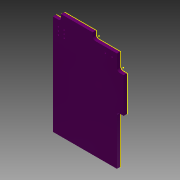
# Autodesk Inventor part: BarePCB
Saved by Autodesk Inventor 2015 SP2 (Build 190223200, 223)
## iProperties
Created: 2016-07-13
Part Number: BarePCB
Material: Generic
Document SubType Name: Modeling
Designer: Iain
Density: 1 g/cm^3
Appearance: Default
Mass: 2.23932 g
Surface Area: 30.5236 cm^2
Volume: 2.23932 cm^3
Author: Iain
Autodesk Inventor part; units mm, degrees
ref_plane "YZ Plane" through (0, 0, 0) normal (1, 0, 0) x (0, 1, 0)
ref_plane "XZ Plane" through (0, 0, 0) normal (0, 1, 0) x (-1, 0, 0)
ref_plane "XY Plane" through (0, 0, 0) normal (0, 0, 1) x (1, 0, 0)
sketch "Sketch1" plane through (0, 0, 0) normal (0, 1, 0) x (-1, 0, 0)
  line L0 (14.5, -22.6) -> (-14.5, -22.6)
  line L1 (-14.5, -22.6) -> (-14.5, 22.6)
  line L2 (-14.5, 22.6) -> (14.5, 22.6)
  line L3 (14.5, 22.6) -> (14.5, -22.6)
  point P0 (0, 0)
  point P1 (0, -22.6)
  point P2 (14.5, 0)
  dimension "d0" = 29
  dimension "d1" = 45.2
  constraints: 8 end point, 2 midpoint, 2 parallel, 1 horizontal, 1 horizontal alignment, 1 perpendicular, 1 vertical alignment
  measures "d0" distance of L0.start L0.end
  measures "d1" distance of L0.end L1.end
extrude "Extrusion1" add sketch "Sketch1" along normal blind 1.6
sketch "Sketch2" plane through (0, 1.6, 0) normal (0, 1, 0) x (1, 0, 0)
  line L0 (14.5, 22.6) -> (-14.5, 22.6) projected
  line L1 (-14.5, 22.6) -> (-14.5, -22.6) projected
  line L2 (-14.5, -22.6) -> (14.5, -22.6) projected
  line L3 (14.5, -22.6) -> (14.5, 22.6) projected
  line L4 (14.5, 0.35) -> (17.5, 0.35)
  line L5 (17.5, 0.35) -> (17.5, -15.6)
  line L6 (17.5, -15.6) -> (14.5, -15.6)
  line L7 (14.5, -15.6) -> (14.5, 0.35)
  point P0 (0, 0)
  point P1 (14.5, -7.625)
  point P2 (14.5, 0)
  dimension "d4" = 3
  dimension "d5" = 15.95
  dimension "d6" = 7
  constraints: 8 end point, 2 midpoint, 2 parallel, 1 horizontal, 1 perpendicular, 1 vertical alignment
  measures "d4" distance of L4.start L4.end
  measures "d5" distance of L4.end L5.end
  measures "d6" distance between parallel lines of L2 L6
extrude "Extrusion2" add sketch "Sketch2" against normal up to surface (1.6 mm away) contours L4 L5 L6 L3
sketch "Sketch3" plane through (0, 1.6, 0) normal (0, 1, 0) x (1, 0, 0)
  line L0 (14.5, 22.6) -> (-14.5, 22.6) projected
  line L1 (-14.5, 22.6) -> (-14.5, -22.6) projected
  line L2 (-14.5, -22.6) -> (14.5, -22.6) projected
  line L3 (14.5, -22.6) -> (14.5, -15.6) projected
  line L4 (17.5, -15.6) -> (14.5, -15.6) projected
  line L5 (17.5, 0.35) -> (17.5, -15.6) projected
  line L6 (14.5, 0.35) -> (17.5, 0.35) projected
  line L7 (14.5, 0.35) -> (14.5, 22.6) projected
  line L8 (-10.8, -22.6) -> (3.5, -22.6)
  line L9 (3.5, -22.6) -> (3.5, -25.4)
  line L10 (3.5, -25.4) -> (-10.8, -25.4)
  line L11 (-10.8, -25.4) -> (-10.8, -22.6)
  line L12 (-14.5, -22.6) -> (14.5, -22.6) projected
  point P0 (0, 0)
  point P1 (-3.65, -22.6)
  point P2 (0, -22.6)
  dimension "d9" = 2.8
  dimension "d10" = 14.3
  dimension "d11" = 3.7
  constraints: 8 end point, 2 midpoint, 2 parallel, 1 horizontal, 1 horizontal alignment, 1 perpendicular
  measures "d9" distance of L8.end L9.end
  measures "d10" distance of L9.end L10.end
  measures "d11" distance between parallel lines of L11 L1
extrude "Extrusion3" add sketch "Sketch3" against normal up to surface (1.6 mm away) contours L2 L9 L10 L11
fillet "Fillet1" radius 1.27 4 edges at (-10.8, 0.8, 22.6) (3.5, 0.8, 22.6) (14.5, 0.8, 15.6) (14.5, 0.8, -0.35)
sketch "Sketch4" plane through (0, 1.6, 0) normal (0, 1, 0) x (1, 0, 0)
  line L0 (14.5, 22.6) -> (-14.5, 22.6) projected
  line L1 (-14.5, 22.6) -> (-14.5, -22.6) projected
  line L2 (-14.5, -22.6) -> (-12.07, -22.6) projected
  arc A0 (-10.8, -23.87) -> (-12.07, -22.6) centre (-12.07, -23.87) ccw projected
  line L3 (-10.8, -25.4) -> (-10.8, -23.87) projected
  line L4 (3.5, -25.4) -> (-10.8, -25.4) projected
  line L5 (3.5, -23.87) -> (3.5, -25.4) projected
  arc A1 (4.77, -22.6) -> (3.5, -23.87) centre (4.77, -23.87) ccw projected
  line L6 (4.77, -22.6) -> (14.5, -22.6) projected
  line L7 (14.5, -22.6) -> (14.5, -16.87) projected
  arc A2 (15.77, -15.6) -> (14.5, -16.87) centre (15.77, -16.87) ccw projected
  line L8 (17.5, -15.6) -> (15.77, -15.6) projected
  line L9 (17.5, 0.35) -> (17.5, -15.6) projected
  line L10 (15.77, 0.35) -> (17.5, 0.35) projected
  arc A3 (14.5, 1.62) -> (15.77, 0.35) centre (15.77, 1.62) ccw projected
  line L11 (14.5, 1.62) -> (14.5, 22.6) projected
  point P0 (0, 0)
  point P1 (12.15, -20.2)
  point P2 (9.15, -20.2)
  dimension "d15" = 2.35
  dimension "d16" = 2.4
  dimension "d17" = 2.4
  dimension "d18" = 5.35
  measures "d15" distance from line of L7 point (12.15, -20.2)
  measures "d16" distance from line of L6 point (12.15, -20.2)
  measures "d17" distance from line of L6 point (9.15, -20.2)
  measures "d18" distance from line of L7 point (9.15, -20.2)
hole "Hole1" at (12.15, 1.6, 20.2) at (9.15, 1.6, 20.2) direction (0, -1, 0) diameter 0.8 end through all
sketch "Sketch5" plane through (0, 1.6, 0) normal (0, 1, 0) x (1, 0, 0)
  circle A0 centre (12.15, -20.2) radius 0.4 projected
  circle A1 centre (9.15, -20.2) radius 0.4 projected
  line L0 (14.5, 22.6) -> (-14.5, 22.6) projected
  line L1 (-14.5, 22.6) -> (-14.5, -22.6) projected
  line L2 (-14.5, -22.6) -> (-12.07, -22.6) projected
  arc A2 (-10.8, -23.87) -> (-12.07, -22.6) centre (-12.07, -23.87) ccw projected
  line L3 (-10.8, -25.4) -> (-10.8, -23.87) projected
  line L4 (3.5, -25.4) -> (-10.8, -25.4) projected
  line L5 (3.5, -23.87) -> (3.5, -25.4) projected
  arc A3 (4.77, -22.6) -> (3.5, -23.87) centre (4.77, -23.87) ccw projected
  line L6 (4.77, -22.6) -> (14.5, -22.6) projected
  line L7 (14.5, -22.6) -> (14.5, -16.87) projected
  arc A4 (15.77, -15.6) -> (14.5, -16.87) centre (15.77, -16.87) ccw projected
  line L8 (17.5, -15.6) -> (15.77, -15.6) projected
  line L9 (17.5, 0.35) -> (17.5, -15.6) projected
  line L10 (15.77, 0.35) -> (17.5, 0.35) projected
  arc A5 (14.5, 1.62) -> (15.77, 0.35) centre (15.77, 1.62) ccw projected
  line L11 (14.5, 1.62) -> (14.5, 22.6) projected
  line L12 (-12.05, -19.95) -> (-12.05, -17) construction
  line L13 (-12.05, -19.95) -> (-11.6759, -19.95) construction
  point P0 (0, 0)
  point P1 (-12.05, -18.35)
  point P2 (-12.05, -16.75)
  point P3 (-9.51, -19.95)
  point P4 (-9.51, -18.35)
  point P5 (-9.51, -16.75)
  dimension "d26" = 2.65
  dimension "d27" = 2.45
  dimension "d30" = 1.6
  dimension "d33" = 2.54
  constraints: 4 end point, 2 horizontal, 2 vertical, 5 other
  measures "d26" distance from line of L2 L12.start
  measures "d27" distance from line of L1 L12.start
  measures "d30" distance of L12.start point (-12.05, -18.35)
  measures "d33" distance of L12.start point (-9.51, -19.95)
hole "Hole2" at (-12.05, 1.6, 19.95) at (-12.05, 1.6, 18.35) at (-12.05, 1.6, 16.75) at (-9.51, 1.6, 19.95) at (-9.51, 1.6, 18.35) at (-9.51, 1.6, 16.75) direction (0, -1, 0) diameter 0.8 end through all
sketch "Sketch6" plane through (0, 1.6, 0) normal (0, 1, 0) x (1, 0, 0)
  circle A0 centre (-9.51, -18.35) radius 0.4 projected
  circle A1 centre (-12.05, -16.75) radius 0.4 projected
  circle A2 centre (-12.05, -19.95) radius 0.4 projected
  circle A3 centre (-12.05, -18.35) radius 0.4 projected
  circle A4 centre (-9.51, -19.95) radius 0.4 projected
  circle A5 centre (-9.51, -16.75) radius 0.4 projected
  circle A6 centre (12.15, -20.2) radius 0.4 projected
  circle A7 centre (9.15, -20.2) radius 0.4 projected
  line L0 (14.5, 22.6) -> (-14.5, 22.6) projected
  line L1 (-14.5, 22.6) -> (-14.5, -22.6) projected
  line L2 (-14.5, -22.6) -> (-12.07, -22.6) projected
  arc A8 (-10.8, -23.87) -> (-12.07, -22.6) centre (-12.07, -23.87) ccw projected
  line L3 (-10.8, -25.4) -> (-10.8, -23.87) projected
  line L4 (3.5, -25.4) -> (-10.8, -25.4) projected
  line L5 (3.5, -23.87) -> (3.5, -25.4) projected
  arc A9 (4.77, -22.6) -> (3.5, -23.87) centre (4.77, -23.87) ccw projected
  line L6 (4.77, -22.6) -> (14.5, -22.6) projected
  line L7 (14.5, -22.6) -> (14.5, -16.87) projected
  arc A10 (15.77, -15.6) -> (14.5, -16.87) centre (15.77, -16.87) ccw projected
  line L8 (17.5, -15.6) -> (15.77, -15.6) projected
  line L9 (17.5, 0.35) -> (17.5, -15.6) projected
  line L10 (15.77, 0.35) -> (17.5, 0.35) projected
  arc A11 (14.5, 1.62) -> (15.77, 0.35) centre (15.77, 1.62) ccw projected
  line L11 (14.5, 1.62) -> (14.5, 22.6) projected
  point P0 (0, 0)
equation "\"d17\" = d16"
body "Solid1"
